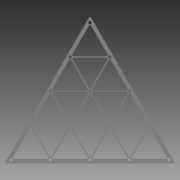
# Autodesk Inventor part: grid16-thin
Saved by Autodesk Inventor 2013 (Build 170138000, 138)
## iProperties
Created: 2013-03-05
Part Number: grid16-thin
Material: Generic
Document SubType Name: Modeling
Designer: Beth Scott
Density: 1 g/cm^3
Author: Beth Scott
Autodesk Inventor part; units mm, degrees
ref_plane "YZ Plane" through (0, 0, 0) normal (1, 0, 0) x (0, 1, 0)
ref_plane "XZ Plane" through (0, 0, 0) normal (0, 1, 0) x (-1, 0, 0)
ref_plane "XY Plane" through (0, 0, 0) normal (0, 0, 1) x (1, 0, 0)
sketch "Triangle 1mm" plane through (0, 0, 0) normal (0, 0, 1) x (1, 0, 0)
  line L0 (0, 0) -> (16.6665, 28.8672) construction
  line L1 (16.6665, 28.8672) -> (33.333, 0) construction
  line L2 (33.333, 0) -> (0, 0) construction
  line L3 (1.7321, 2) -> (15.8005, 26.3672)
  line L4 (17.5325, 26.3672) -> (31.6009, 2)
  line L5 (30.7349, 0.5) -> (2.5981, 0.5)
  arc A0 (17.5325, 26.3672) -> (15.8005, 26.3672) centre (16.6665, 25.8672) ccw
  arc A1 (30.7349, 0.5) -> (31.6009, 2) centre (30.7349, 1.5) ccw
  arc A2 (1.7321, 2) -> (2.5981, 0.5) centre (2.5981, 1.5) ccw
  line L6 (33.333, 0) -> (8.3332, 14.4336) construction
  line L7 (0, 0) -> (24.9997, 14.4336) construction
  line L8 (16.6665, 28.8672) -> (16.6665, 0) construction
  point P0 (16.9666, 9.7956)
  dimension "d14" = 33.333
  dimension "d17" = 1
  dimension "d18" = 0.5
  measures "d14" distance of L1.end L0.start
  measures "d17" radius of A2
  measures "d18" distance from line of L4 L7.end
sketch "Tri16 1mm" plane through (0, 0, 0) normal (0, 0, 1) x (1, 0, 0)
  line L0 (0, 0) -> (16.6665, 28.8672) construction
  line L1 (16.6665, 28.8672) -> (33.333, 0) construction
  line L2 (33.333, 0) -> (0, 0) construction
  line L3 (1.7321, 2) -> (15.8005, 26.3672)
  line L4 (17.5325, 26.3672) -> (31.6009, 2)
  line L5 (30.7349, 0.5) -> (2.5981, 0.5)
  arc A0 (17.5325, 26.3672) -> (15.8005, 26.3672) centre (16.6665, 25.8672) ccw
  arc A1 (30.7349, 0.5) -> (31.6009, 2) centre (30.7349, 1.5) ccw
  arc A2 (1.7321, 2) -> (2.5981, 0.5) centre (2.5981, 1.5) ccw
  line L6 (33.333, 0) -> (8.3333, 14.4336) construction
  line L7 (0, 0) -> (24.9998, 14.4336) construction
  line L8 (16.6665, 28.8672) -> (16.6665, 0) construction
  line L9 (33.333, 0) -> (49.9995, 28.8672) construction
  line L10 (49.9995, 28.8672) -> (66.666, 0) construction
  line L11 (66.666, 0) -> (33.333, 0) construction
  line L12 (35.0651, 2) -> (49.1335, 26.3672)
  line L13 (50.8655, 26.3672) -> (64.9339, 2)
  line L14 (64.0679, 0.5) -> (35.9311, 0.5)
  arc A3 (50.8655, 26.3672) -> (49.1335, 26.3672) centre (49.9995, 25.8672) ccw
  arc A4 (64.0679, 0.5) -> (64.9339, 2) centre (64.0679, 1.5) ccw
  arc A5 (35.0651, 2) -> (35.9311, 0.5) centre (35.9311, 1.5) ccw
  line L15 (66.666, 0) -> (41.6663, 14.4336) construction
  line L16 (33.333, 0) -> (58.3328, 14.4336) construction
  line L17 (49.9995, 28.8672) -> (49.9995, 0) construction
  line L18 (49.9995, 28.8672) -> (33.333, 0) construction
  line L19 (33.333, 0) -> (16.6665, 28.8672) construction
  line L20 (16.6665, 28.8672) -> (49.9995, 28.8672) construction
  line L21 (48.2674, 26.8672) -> (34.199, 2.5)
  line L22 (32.467, 2.5) -> (18.3986, 26.8672)
  line L23 (19.2646, 28.3672) -> (47.4014, 28.3672)
  arc A6 (32.467, 2.5) -> (34.199, 2.5) centre (33.333, 3) ccw
  arc A7 (19.2646, 28.3672) -> (18.3986, 26.8672) centre (19.2646, 27.3672) ccw
  arc A8 (48.2674, 26.8672) -> (47.4014, 28.3672) centre (47.4014, 27.3672) ccw
  line L24 (16.6665, 28.8672) -> (41.6663, 14.4336) construction
  line L25 (49.9995, 28.8672) -> (24.9998, 14.4336) construction
  line L26 (33.333, 0) -> (33.333, 28.8672) construction
  line L27 (83.3325, 28.8672) -> (66.666, 0) construction
  line L28 (66.666, 0) -> (49.9995, 28.8672) construction
  line L29 (49.9995, 28.8672) -> (83.3325, 28.8672) construction
  line L30 (81.6004, 26.8672) -> (67.532, 2.5)
  line L31 (65.8, 2.5) -> (51.7316, 26.8672)
  line L32 (52.5976, 28.3672) -> (80.7344, 28.3672)
  arc A9 (65.8, 2.5) -> (67.532, 2.5) centre (66.666, 3) ccw
  arc A10 (52.5976, 28.3672) -> (51.7316, 26.8672) centre (52.5976, 27.3672) ccw
  arc A11 (81.6004, 26.8672) -> (80.7344, 28.3672) centre (80.7344, 27.3672) ccw
  line L33 (49.9995, 28.8672) -> (74.9993, 14.4336) construction
  line L34 (83.3325, 28.8672) -> (58.3328, 14.4336) construction
  line L35 (66.666, 0) -> (66.666, 28.8672) construction
  line L36 (66.666, 0) -> (83.3325, 28.8672) construction
  line L37 (83.3325, 28.8672) -> (99.999, 0) construction
  line L38 (99.999, 0) -> (66.666, 0) construction
  line L39 (68.3981, 2) -> (82.4665, 26.3672)
  line L40 (84.1985, 26.3672) -> (98.2669, 2)
  line L41 (97.4009, 0.5) -> (69.2641, 0.5)
  arc A12 (84.1985, 26.3672) -> (82.4665, 26.3672) centre (83.3325, 25.8672) ccw
  arc A13 (97.4009, 0.5) -> (98.2669, 2) centre (97.4009, 1.5) ccw
  arc A14 (68.3981, 2) -> (69.2641, 0.5) centre (69.2641, 1.5) ccw
  line L42 (99.999, 0) -> (74.9993, 14.4336) construction
  line L43 (66.666, 0) -> (91.6658, 14.4336) construction
  line L44 (83.3325, 28.8672) -> (83.3325, 0) construction
  line L45 (99.999, 0) -> (116.6655, 28.8672) construction
  line L46 (116.6655, 28.8672) -> (133.332, 0) construction
  line L47 (133.332, 0) -> (99.999, 0) construction
  line L48 (101.7311, 2) -> (115.7995, 26.3672)
  line L49 (117.5315, 26.3672) -> (131.5999, 2)
  line L50 (130.7339, 0.5) -> (102.5971, 0.5)
  arc A15 (117.5315, 26.3672) -> (115.7995, 26.3672) centre (116.6655, 25.8672) ccw
  arc A16 (130.7339, 0.5) -> (131.5999, 2) centre (130.7339, 1.5) ccw
  arc A17 (101.7311, 2) -> (102.5971, 0.5) centre (102.5971, 1.5) ccw
  line L51 (133.332, 0) -> (108.3323, 14.4336) construction
  line L52 (99.999, 0) -> (124.9988, 14.4336) construction
  line L53 (116.6655, 28.8672) -> (116.6655, 0) construction
  line L54 (116.6655, 28.8672) -> (99.999, 0) construction
  line L55 (99.999, 0) -> (83.3325, 28.8672) construction
  line L56 (83.3325, 28.8672) -> (116.6655, 28.8672) construction
  line L57 (114.9334, 26.8672) -> (100.865, 2.5)
  line L58 (99.133, 2.5) -> (85.0646, 26.8672)
  line L59 (85.9306, 28.3672) -> (114.0674, 28.3672)
  arc A18 (99.133, 2.5) -> (100.865, 2.5) centre (99.999, 3) ccw
  arc A19 (85.9306, 28.3672) -> (85.0646, 26.8672) centre (85.9306, 27.3672) ccw
  arc A20 (114.9334, 26.8672) -> (114.0674, 28.3672) centre (114.0674, 27.3672) ccw
  line L60 (83.3325, 28.8672) -> (108.3323, 14.4336) construction
  line L61 (116.6655, 28.8672) -> (91.6658, 14.4336) construction
  line L62 (99.999, 0) -> (99.999, 28.8672) construction
  line L63 (16.6665, 28.8672) -> (33.333, 57.7344) construction
  line L64 (33.333, 57.7344) -> (49.9995, 28.8672) construction
  line L65 (49.9995, 28.8672) -> (16.6665, 28.8672) construction
  line L66 (18.3986, 30.8672) -> (32.467, 55.2344)
  line L67 (34.199, 55.2344) -> (48.2674, 30.8672)
  line L68 (47.4014, 29.3672) -> (19.2646, 29.3672)
  arc A21 (34.199, 55.2344) -> (32.467, 55.2344) centre (33.333, 54.7344) ccw
  arc A22 (47.4014, 29.3672) -> (48.2674, 30.8672) centre (47.4014, 30.3672) ccw
  arc A23 (18.3986, 30.8672) -> (19.2646, 29.3672) centre (19.2646, 30.3672) ccw
  line L69 (49.9995, 28.8672) -> (24.9998, 43.3008) construction
  line L70 (16.6665, 28.8672) -> (41.6663, 43.3008) construction
  line L71 (33.333, 57.7344) -> (33.333, 28.8672) construction
  line L72 (33.333, 57.7344) -> (49.9995, 86.6017) construction
  line L73 (49.9995, 86.6017) -> (66.666, 57.7344) construction
  line L74 (66.666, 57.7344) -> (33.333, 57.7344) construction
  line L75 (35.0651, 59.7344) -> (49.1335, 84.1017)
  line L76 (50.8655, 84.1017) -> (64.9339, 59.7344)
  line L77 (64.0679, 58.2344) -> (35.9311, 58.2344)
  arc A24 (50.8655, 84.1017) -> (49.1335, 84.1017) centre (49.9995, 83.6017) ccw
  arc A25 (64.0679, 58.2344) -> (64.9339, 59.7344) centre (64.0679, 59.2344) ccw
  arc A26 (35.0651, 59.7344) -> (35.9311, 58.2344) centre (35.9311, 59.2344) ccw
  line L78 (66.666, 57.7344) -> (41.6663, 72.1681) construction
  line L79 (33.333, 57.7344) -> (58.3328, 72.1681) construction
  line L80 (49.9995, 86.6017) -> (49.9995, 57.7344) construction
  line L81 (49.9995, 86.6017) -> (66.666, 115.4689) construction
  line L82 (66.666, 115.4689) -> (83.3325, 86.6017) construction
  line L83 (83.3325, 86.6017) -> (49.9995, 86.6017) construction
  line L84 (51.7316, 88.6017) -> (65.8, 112.9689)
  line L85 (67.532, 112.9689) -> (81.6004, 88.6017)
  line L86 (80.7344, 87.1017) -> (52.5976, 87.1017)
  arc A27 (67.532, 112.9689) -> (65.8, 112.9689) centre (66.666, 112.4689) ccw
  arc A28 (80.7344, 87.1017) -> (81.6004, 88.6017) centre (80.7344, 88.1017) ccw
  arc A29 (51.7316, 88.6017) -> (52.5976, 87.1017) centre (52.5976, 88.1017) ccw
  line L87 (83.3325, 86.6017) -> (58.3328, 101.0353) construction
  line L88 (49.9995, 86.6017) -> (74.9993, 101.0353) construction
  line L89 (66.666, 115.4689) -> (66.666, 86.6017) construction
  line L90 (66.666, 57.7344) -> (49.9995, 28.8672) construction
  line L91 (49.9995, 28.8672) -> (33.333, 57.7344) construction
  line L92 (33.333, 57.7344) -> (66.666, 57.7344) construction
  line L93 (64.9339, 55.7344) -> (50.8655, 31.3672)
  line L94 (49.1335, 31.3672) -> (35.0651, 55.7344)
  line L95 (35.9311, 57.2344) -> (64.0679, 57.2344)
  arc A30 (49.1335, 31.3672) -> (50.8655, 31.3672) centre (49.9995, 31.8672) ccw
  arc A31 (35.9311, 57.2344) -> (35.0651, 55.7344) centre (35.9311, 56.2344) ccw
  arc A32 (64.9339, 55.7344) -> (64.0679, 57.2344) centre (64.0679, 56.2344) ccw
  line L96 (33.333, 57.7344) -> (58.3328, 43.3008) construction
  line L97 (66.666, 57.7344) -> (41.6663, 43.3008) construction
  line L98 (49.9995, 28.8672) -> (49.9995, 57.7344) construction
  line L99 (83.3325, 86.6017) -> (66.666, 57.7344) construction
  line L100 (66.666, 57.7344) -> (49.9995, 86.6017) construction
  line L101 (49.9995, 86.6017) -> (83.3325, 86.6017) construction
  line L102 (81.6004, 84.6017) -> (67.532, 60.2344)
  line L103 (65.8, 60.2344) -> (51.7316, 84.6017)
  line L104 (52.5976, 86.1017) -> (80.7344, 86.1017)
  arc A33 (65.8, 60.2344) -> (67.532, 60.2344) centre (66.666, 60.7344) ccw
  arc A34 (52.5976, 86.1017) -> (51.7316, 84.6017) centre (52.5976, 85.1017) ccw
  arc A35 (81.6004, 84.6017) -> (80.7344, 86.1017) centre (80.7344, 85.1017) ccw
  line L105 (49.9995, 86.6017) -> (74.9993, 72.1681) construction
  line L106 (83.3325, 86.6017) -> (58.3328, 72.1681) construction
  line L107 (66.666, 57.7344) -> (66.666, 86.6017) construction
  line L108 (66.666, 57.7344) -> (83.3325, 86.6017) construction
  line L109 (83.3325, 86.6017) -> (99.999, 57.7344) construction
  line L110 (99.999, 57.7344) -> (66.666, 57.7344) construction
  line L111 (68.3981, 59.7344) -> (82.4665, 84.1017)
  line L112 (84.1985, 84.1017) -> (98.2669, 59.7344)
  line L113 (97.4009, 58.2344) -> (69.2641, 58.2344)
  arc A36 (84.1985, 84.1017) -> (82.4665, 84.1017) centre (83.3325, 83.6017) ccw
  arc A37 (97.4009, 58.2344) -> (98.2669, 59.7344) centre (97.4009, 59.2344) ccw
  arc A38 (68.3981, 59.7344) -> (69.2641, 58.2344) centre (69.2641, 59.2344) ccw
  line L114 (99.999, 57.7344) -> (74.9993, 72.1681) construction
  line L115 (66.666, 57.7344) -> (91.6658, 72.1681) construction
  line L116 (83.3325, 86.6017) -> (83.3325, 57.7344) construction
  line L117 (49.9995, 28.8672) -> (66.666, 57.7344) construction
  line L118 (66.666, 57.7344) -> (83.3325, 28.8672) construction
  line L119 (83.3325, 28.8672) -> (49.9995, 28.8672) construction
  line L120 (51.7316, 30.8672) -> (65.8, 55.2344)
  line L121 (67.532, 55.2344) -> (81.6004, 30.8672)
  line L122 (80.7344, 29.3672) -> (52.5976, 29.3672)
  arc A39 (67.532, 55.2344) -> (65.8, 55.2344) centre (66.666, 54.7344) ccw
  arc A40 (80.7344, 29.3672) -> (81.6004, 30.8672) centre (80.7344, 30.3672) ccw
  arc A41 (51.7316, 30.8672) -> (52.5976, 29.3672) centre (52.5976, 30.3672) ccw
  line L123 (83.3325, 28.8672) -> (58.3328, 43.3008) construction
  line L124 (49.9995, 28.8672) -> (74.9993, 43.3008) construction
  line L125 (66.666, 57.7344) -> (66.666, 28.8672) construction
  line L126 (83.3325, 28.8672) -> (99.999, 57.7344) construction
  line L127 (99.999, 57.7344) -> (116.6655, 28.8672) construction
  line L128 (116.6655, 28.8672) -> (83.3325, 28.8672) construction
  line L129 (85.0646, 30.8672) -> (99.133, 55.2344)
  line L130 (100.865, 55.2344) -> (114.9334, 30.8672)
  line L131 (114.0674, 29.3672) -> (85.9306, 29.3672)
  arc A42 (100.865, 55.2344) -> (99.133, 55.2344) centre (99.999, 54.7344) ccw
  arc A43 (114.0674, 29.3672) -> (114.9334, 30.8672) centre (114.0674, 30.3672) ccw
  arc A44 (85.0646, 30.8672) -> (85.9306, 29.3672) centre (85.9306, 30.3672) ccw
  line L132 (116.6655, 28.8672) -> (91.6658, 43.3008) construction
  line L133 (83.3325, 28.8672) -> (108.3323, 43.3008) construction
  line L134 (99.999, 57.7344) -> (99.999, 28.8672) construction
  line L135 (99.999, 57.7344) -> (83.3325, 28.8672) construction
  line L136 (83.3325, 28.8672) -> (66.666, 57.7344) construction
  line L137 (66.666, 57.7344) -> (99.999, 57.7344) construction
  line L138 (98.2669, 55.7344) -> (84.1985, 31.3672)
  line L139 (82.4665, 31.3672) -> (68.3981, 55.7344)
  line L140 (69.2641, 57.2344) -> (97.4009, 57.2344)
  arc A45 (82.4665, 31.3672) -> (84.1985, 31.3672) centre (83.3325, 31.8672) ccw
  arc A46 (69.2641, 57.2344) -> (68.3981, 55.7344) centre (69.2641, 56.2344) ccw
  arc A47 (98.2669, 55.7344) -> (97.4009, 57.2344) centre (97.4009, 56.2344) ccw
  line L141 (66.666, 57.7344) -> (91.6658, 43.3008) construction
  line L142 (99.999, 57.7344) -> (74.9993, 43.3008) construction
  line L143 (83.3325, 28.8672) -> (83.3325, 57.7344) construction
  point P0 (66.741, 38.5329)
sketch "Top Plate" plane through (0, 0, 0) normal (0, 1, 0) x (-1, 0, 0)
  line L0 (-4.3301, -1.5) -> (65.8, 119.9689)
  line L1 (67.532, 119.9689) -> (137.6621, -1.5)
  line L2 (-3.4641, -3) -> (136.7961, -3)
  circle A0 centre (33.333, 0) radius 1.5
  circle A1 centre (0, 0) radius 1.5
  circle A2 centre (16.6665, 28.8672) radius 1.5
  circle A3 centre (33.333, 57.7344) radius 1.5
  circle A4 centre (49.9995, 28.8672) radius 1.5
  circle A5 centre (66.666, 0) radius 1.5
  circle A6 centre (99.999, 0) radius 1.5
  circle A7 centre (133.332, 0) radius 1.5
  circle A8 centre (116.6655, 28.8672) radius 1.5
  circle A9 centre (99.999, 57.7344) radius 1.5
  circle A10 centre (83.3325, 28.8672) radius 1.5
  circle A11 centre (66.666, 57.7344) radius 1.5
  circle A12 centre (83.3325, 86.6017) radius 1.5
  circle A13 centre (49.9995, 86.6017) radius 1.5
  circle A14 centre (66.666, 115.4689) radius 1.5
  arc A15 (67.532, 119.9689) -> (65.8, 119.9689) centre (66.666, 119.4689) ccw
  arc A16 (136.7961, -3) -> (137.6621, -1.5) centre (136.7961, -2) ccw
  arc A17 (-4.3301, -1.5) -> (-3.4641, -3) centre (-3.4641, -2) ccw
  line L3 (0, 0) -> (-13.8976, -8.0238) construction
  line L4 (133.332, 0) -> (144.2364, -6.2956) construction
  circle A18 centre (16.6665, 28.8672) radius 3 construction
  line L5 (0, 0) -> (16.6665, 28.8672) construction
  line L6 (16.6665, 28.8672) -> (33.333, 0) construction
  line L7 (33.333, 0) -> (0, 0) construction
  line L8 (1.7321, 2) -> (15.8005, 26.3672)
  line L9 (17.5325, 26.3672) -> (31.6009, 2)
  line L10 (30.7349, 0.5) -> (2.5981, 0.5)
  arc A19 (17.5325, 26.3672) -> (15.8005, 26.3672) centre (16.6665, 25.8672) ccw
  arc A20 (30.7349, 0.5) -> (31.6009, 2) centre (30.7349, 1.5) ccw
  arc A21 (1.7321, 2) -> (2.5981, 0.5) centre (2.5981, 1.5) ccw
  line L11 (33.333, 0) -> (8.3333, 14.4336) construction
  line L12 (0, 0) -> (24.9998, 14.4336) construction
  line L13 (16.6665, 28.8672) -> (16.6665, 0) construction
  line L14 (33.333, 0) -> (49.9995, 28.8672) construction
  line L15 (49.9995, 28.8672) -> (66.666, 0) construction
  line L16 (66.666, 0) -> (33.333, 0) construction
  line L17 (35.0651, 2) -> (49.1335, 26.3672)
  line L18 (50.8655, 26.3672) -> (64.9339, 2)
  line L19 (64.0679, 0.5) -> (35.9311, 0.5)
  arc A22 (50.8655, 26.3672) -> (49.1335, 26.3672) centre (49.9995, 25.8672) ccw
  arc A23 (64.0679, 0.5) -> (64.9339, 2) centre (64.0679, 1.5) ccw
  arc A24 (35.0651, 2) -> (35.9311, 0.5) centre (35.9311, 1.5) ccw
  line L20 (66.666, 0) -> (41.6663, 14.4336) construction
  line L21 (33.333, 0) -> (58.3328, 14.4336) construction
  line L22 (49.9995, 28.8672) -> (49.9995, 0) construction
  line L23 (49.9995, 28.8672) -> (33.333, 0) construction
  line L24 (33.333, 0) -> (16.6665, 28.8672) construction
  line L25 (16.6665, 28.8672) -> (49.9995, 28.8672) construction
  line L26 (48.2674, 26.8672) -> (34.199, 2.5)
  line L27 (32.467, 2.5) -> (18.3986, 26.8672)
  line L28 (19.2646, 28.3672) -> (47.4014, 28.3672)
  arc A25 (32.467, 2.5) -> (34.199, 2.5) centre (33.333, 3) ccw
  arc A26 (19.2646, 28.3672) -> (18.3986, 26.8672) centre (19.2646, 27.3672) ccw
  arc A27 (48.2674, 26.8672) -> (47.4014, 28.3672) centre (47.4014, 27.3672) ccw
  line L29 (16.6665, 28.8672) -> (41.6663, 14.4336) construction
  line L30 (49.9995, 28.8672) -> (24.9998, 14.4336) construction
  line L31 (33.333, 0) -> (33.333, 28.8672) construction
  line L32 (83.3325, 28.8672) -> (66.666, 0) construction
  line L33 (66.666, 0) -> (49.9995, 28.8672) construction
  line L34 (49.9995, 28.8672) -> (83.3325, 28.8672) construction
  line L35 (81.6004, 26.8672) -> (67.532, 2.5)
  line L36 (65.8, 2.5) -> (51.7316, 26.8672)
  line L37 (52.5976, 28.3672) -> (80.7344, 28.3672)
  arc A28 (65.8, 2.5) -> (67.532, 2.5) centre (66.666, 3) ccw
  arc A29 (52.5976, 28.3672) -> (51.7316, 26.8672) centre (52.5976, 27.3672) ccw
  arc A30 (81.6004, 26.8672) -> (80.7344, 28.3672) centre (80.7344, 27.3672) ccw
  line L38 (49.9995, 28.8672) -> (74.9993, 14.4336) construction
  line L39 (83.3325, 28.8672) -> (58.3328, 14.4336) construction
  line L40 (66.666, 0) -> (66.666, 28.8672) construction
  line L41 (66.666, 0) -> (83.3325, 28.8672) construction
  line L42 (83.3325, 28.8672) -> (99.999, 0) construction
  line L43 (99.999, 0) -> (66.666, 0) construction
  line L44 (68.3981, 2) -> (82.4665, 26.3672)
  line L45 (84.1985, 26.3672) -> (98.2669, 2)
  line L46 (97.4009, 0.5) -> (69.2641, 0.5)
  arc A31 (84.1985, 26.3672) -> (82.4665, 26.3672) centre (83.3325, 25.8672) ccw
  arc A32 (97.4009, 0.5) -> (98.2669, 2) centre (97.4009, 1.5) ccw
  arc A33 (68.3981, 2) -> (69.2641, 0.5) centre (69.2641, 1.5) ccw
  line L47 (99.999, 0) -> (74.9993, 14.4336) construction
  line L48 (66.666, 0) -> (91.6658, 14.4336) construction
  line L49 (83.3325, 28.8672) -> (83.3325, 0) construction
  line L50 (99.999, 0) -> (116.6655, 28.8672) construction
  line L51 (116.6655, 28.8672) -> (133.332, 0) construction
  line L52 (133.332, 0) -> (99.999, 0) construction
  line L53 (101.7311, 2) -> (115.7995, 26.3672)
  line L54 (117.5315, 26.3672) -> (131.5999, 2)
  line L55 (130.7339, 0.5) -> (102.5971, 0.5)
  arc A34 (117.5315, 26.3672) -> (115.7995, 26.3672) centre (116.6655, 25.8672) ccw
  arc A35 (130.7339, 0.5) -> (131.5999, 2) centre (130.7339, 1.5) ccw
  arc A36 (101.7311, 2) -> (102.5971, 0.5) centre (102.5971, 1.5) ccw
  line L56 (133.332, 0) -> (108.3323, 14.4336) construction
  line L57 (99.999, 0) -> (124.9988, 14.4336) construction
  line L58 (116.6655, 28.8672) -> (116.6655, 0) construction
  line L59 (116.6655, 28.8672) -> (99.999, 0) construction
  line L60 (99.999, 0) -> (83.3325, 28.8672) construction
  line L61 (83.3325, 28.8672) -> (116.6655, 28.8672) construction
  line L62 (114.9334, 26.8672) -> (100.865, 2.5)
  line L63 (99.133, 2.5) -> (85.0646, 26.8672)
  line L64 (85.9306, 28.3672) -> (114.0674, 28.3672)
  arc A37 (99.133, 2.5) -> (100.865, 2.5) centre (99.999, 3) ccw
  arc A38 (85.9306, 28.3672) -> (85.0646, 26.8672) centre (85.9306, 27.3672) ccw
  arc A39 (114.9334, 26.8672) -> (114.0674, 28.3672) centre (114.0674, 27.3672) ccw
  line L65 (83.3325, 28.8672) -> (108.3323, 14.4336) construction
  line L66 (116.6655, 28.8672) -> (91.6658, 14.4336) construction
  line L67 (99.999, 0) -> (99.999, 28.8672) construction
  line L68 (16.6665, 28.8672) -> (33.333, 57.7344) construction
  line L69 (33.333, 57.7344) -> (49.9995, 28.8672) construction
  line L70 (49.9995, 28.8672) -> (16.6665, 28.8672) construction
  line L71 (18.3986, 30.8672) -> (32.467, 55.2344)
  line L72 (34.199, 55.2344) -> (48.2674, 30.8672)
  line L73 (47.4014, 29.3672) -> (19.2646, 29.3672)
  arc A40 (34.199, 55.2344) -> (32.467, 55.2344) centre (33.333, 54.7344) ccw
  arc A41 (47.4014, 29.3672) -> (48.2674, 30.8672) centre (47.4014, 30.3672) ccw
  arc A42 (18.3986, 30.8672) -> (19.2646, 29.3672) centre (19.2646, 30.3672) ccw
  line L74 (49.9995, 28.8672) -> (24.9998, 43.3008) construction
  line L75 (16.6665, 28.8672) -> (41.6663, 43.3008) construction
  line L76 (33.333, 57.7344) -> (33.333, 28.8672) construction
  line L77 (33.333, 57.7344) -> (49.9995, 86.6017) construction
  line L78 (49.9995, 86.6017) -> (66.666, 57.7344) construction
  line L79 (66.666, 57.7344) -> (33.333, 57.7344) construction
  line L80 (35.0651, 59.7344) -> (49.1335, 84.1017)
  line L81 (50.8655, 84.1017) -> (64.9339, 59.7344)
  line L82 (64.0679, 58.2344) -> (35.9311, 58.2344)
  arc A43 (50.8655, 84.1017) -> (49.1335, 84.1017) centre (49.9995, 83.6017) ccw
  arc A44 (64.0679, 58.2344) -> (64.9339, 59.7344) centre (64.0679, 59.2344) ccw
  arc A45 (35.0651, 59.7344) -> (35.9311, 58.2344) centre (35.9311, 59.2344) ccw
  line L83 (66.666, 57.7344) -> (41.6663, 72.1681) construction
  line L84 (33.333, 57.7344) -> (58.3328, 72.1681) construction
  line L85 (49.9995, 86.6017) -> (49.9995, 57.7344) construction
  line L86 (49.9995, 86.6017) -> (66.666, 115.4689) construction
  line L87 (66.666, 115.4689) -> (83.3325, 86.6017) construction
  line L88 (83.3325, 86.6017) -> (49.9995, 86.6017) construction
  line L89 (51.7316, 88.6017) -> (65.8, 112.9689)
  line L90 (67.532, 112.9689) -> (81.6004, 88.6017)
  line L91 (80.7344, 87.1017) -> (52.5976, 87.1017)
  arc A46 (67.532, 112.9689) -> (65.8, 112.9689) centre (66.666, 112.4689) ccw
  arc A47 (80.7344, 87.1017) -> (81.6004, 88.6017) centre (80.7344, 88.1017) ccw
  arc A48 (51.7316, 88.6017) -> (52.5976, 87.1017) centre (52.5976, 88.1017) ccw
  line L92 (83.3325, 86.6017) -> (58.3328, 101.0353) construction
  line L93 (49.9995, 86.6017) -> (74.9993, 101.0353) construction
  line L94 (66.666, 115.4689) -> (66.666, 86.6017) construction
  line L95 (66.666, 57.7344) -> (49.9995, 28.8672) construction
  line L96 (49.9995, 28.8672) -> (33.333, 57.7344) construction
  line L97 (33.333, 57.7344) -> (66.666, 57.7344) construction
  line L98 (64.9339, 55.7344) -> (50.8655, 31.3672)
  line L99 (49.1335, 31.3672) -> (35.0651, 55.7344)
  line L100 (35.9311, 57.2344) -> (64.0679, 57.2344)
  arc A49 (49.1335, 31.3672) -> (50.8655, 31.3672) centre (49.9995, 31.8672) ccw
  arc A50 (35.9311, 57.2344) -> (35.0651, 55.7344) centre (35.9311, 56.2344) ccw
  arc A51 (64.9339, 55.7344) -> (64.0679, 57.2344) centre (64.0679, 56.2344) ccw
  line L101 (33.333, 57.7344) -> (58.3328, 43.3008) construction
  line L102 (66.666, 57.7344) -> (41.6663, 43.3008) construction
  line L103 (49.9995, 28.8672) -> (49.9995, 57.7344) construction
  line L104 (83.3325, 86.6017) -> (66.666, 57.7344) construction
  line L105 (66.666, 57.7344) -> (49.9995, 86.6017) construction
  line L106 (49.9995, 86.6017) -> (83.3325, 86.6017) construction
  line L107 (81.6004, 84.6017) -> (67.532, 60.2344)
  line L108 (65.8, 60.2344) -> (51.7316, 84.6017)
  line L109 (52.5976, 86.1017) -> (80.7344, 86.1017)
  arc A52 (65.8, 60.2344) -> (67.532, 60.2344) centre (66.666, 60.7344) ccw
  arc A53 (52.5976, 86.1017) -> (51.7316, 84.6017) centre (52.5976, 85.1017) ccw
  arc A54 (81.6004, 84.6017) -> (80.7344, 86.1017) centre (80.7344, 85.1017) ccw
  line L110 (49.9995, 86.6017) -> (74.9993, 72.1681) construction
  line L111 (83.3325, 86.6017) -> (58.3328, 72.1681) construction
  line L112 (66.666, 57.7344) -> (66.666, 86.6017) construction
  line L113 (66.666, 57.7344) -> (83.3325, 86.6017) construction
  line L114 (83.3325, 86.6017) -> (99.999, 57.7344) construction
  line L115 (99.999, 57.7344) -> (66.666, 57.7344) construction
  line L116 (68.3981, 59.7344) -> (82.4665, 84.1017)
  line L117 (84.1985, 84.1017) -> (98.2669, 59.7344)
  line L118 (97.4009, 58.2344) -> (69.2641, 58.2344)
  arc A55 (84.1985, 84.1017) -> (82.4665, 84.1017) centre (83.3325, 83.6017) ccw
  arc A56 (97.4009, 58.2344) -> (98.2669, 59.7344) centre (97.4009, 59.2344) ccw
  arc A57 (68.3981, 59.7344) -> (69.2641, 58.2344) centre (69.2641, 59.2344) ccw
  line L119 (99.999, 57.7344) -> (74.9993, 72.1681) construction
  line L120 (66.666, 57.7344) -> (91.6658, 72.1681) construction
  line L121 (83.3325, 86.6017) -> (83.3325, 57.7344) construction
  line L122 (49.9995, 28.8672) -> (66.666, 57.7344) construction
  line L123 (66.666, 57.7344) -> (83.3325, 28.8672) construction
  line L124 (83.3325, 28.8672) -> (49.9995, 28.8672) construction
  line L125 (51.7316, 30.8672) -> (65.8, 55.2344)
  line L126 (67.532, 55.2344) -> (81.6004, 30.8672)
  line L127 (80.7344, 29.3672) -> (52.5976, 29.3672)
  arc A58 (67.532, 55.2344) -> (65.8, 55.2344) centre (66.666, 54.7344) ccw
  arc A59 (80.7344, 29.3672) -> (81.6004, 30.8672) centre (80.7344, 30.3672) ccw
  arc A60 (51.7316, 30.8672) -> (52.5976, 29.3672) centre (52.5976, 30.3672) ccw
  line L128 (83.3325, 28.8672) -> (58.3328, 43.3008) construction
  line L129 (49.9995, 28.8672) -> (74.9993, 43.3008) construction
  line L130 (66.666, 57.7344) -> (66.666, 28.8672) construction
  line L131 (83.3325, 28.8672) -> (99.999, 57.7344) construction
  line L132 (99.999, 57.7344) -> (116.6655, 28.8672) construction
  line L133 (116.6655, 28.8672) -> (83.3325, 28.8672) construction
  line L134 (85.0646, 30.8672) -> (99.133, 55.2344)
  line L135 (100.865, 55.2344) -> (114.9334, 30.8672)
  line L136 (114.0674, 29.3672) -> (85.9306, 29.3672)
  arc A61 (100.865, 55.2344) -> (99.133, 55.2344) centre (99.999, 54.7344) ccw
  arc A62 (114.0674, 29.3672) -> (114.9334, 30.8672) centre (114.0674, 30.3672) ccw
  arc A63 (85.0646, 30.8672) -> (85.9306, 29.3672) centre (85.9306, 30.3672) ccw
  line L137 (116.6655, 28.8672) -> (91.6658, 43.3008) construction
  line L138 (83.3325, 28.8672) -> (108.3323, 43.3008) construction
  line L139 (99.999, 57.7344) -> (99.999, 28.8672) construction
  line L140 (99.999, 57.7344) -> (83.3325, 28.8672) construction
  line L141 (83.3325, 28.8672) -> (66.666, 57.7344) construction
  line L142 (66.666, 57.7344) -> (99.999, 57.7344) construction
  line L143 (98.2669, 55.7344) -> (84.1985, 31.3672)
  line L144 (82.4665, 31.3672) -> (68.3981, 55.7344)
  line L145 (69.2641, 57.2344) -> (97.4009, 57.2344)
  arc A64 (82.4665, 31.3672) -> (84.1985, 31.3672) centre (83.3325, 31.8672) ccw
  arc A65 (69.2641, 57.2344) -> (68.3981, 55.7344) centre (69.2641, 56.2344) ccw
  arc A66 (98.2669, 55.7344) -> (97.4009, 57.2344) centre (97.4009, 56.2344) ccw
  line L146 (66.666, 57.7344) -> (91.6658, 43.3008) construction
  line L147 (99.999, 57.7344) -> (74.9993, 43.3008) construction
  line L148 (83.3325, 28.8672) -> (83.3325, 57.7344) construction
  dimension "d25" = 3
  dimension "d32" = 6
  constraints: 19 centre point, 14 equal radius, 10 end point, 7 tangent, 6 point on circle, 2 point on line, 1 coincident, 1 horizontal, 22 other
  measures "d25" diameter of A0
  measures "d32" diameter of A18
extrude "Top Plate extrusion" add sketch "Top Plate" along normal blind 1.5875
body "Solid2"
